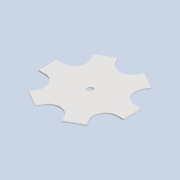
# Autodesk Inventor part: mid_7mm
Saved by Autodesk Inventor 2020 (Build 240168000, 168)
## iProperties
Created: 2021-10-03
Part Number: mid_7mm
Material: Generic
Document SubType Name: Modeling
Designer: Shuang Peng
Density: 1 g/cm^3
Appearance: Default
Author: Shuang Peng
Autodesk Inventor part; units mm, degrees
ref_plane "YZ Plane" through (0, 0, 0) normal (1, 0, 0) x (0, 1, 0)
ref_plane "XZ Plane" through (0, 0, 0) normal (0, 1, 0) x (-1, 0, 0)
ref_plane "XY Plane" through (0, 0, 0) normal (0, 0, 1) x (1, 0, 0)
sketch "Sketch1" plane through (0, 0, 0) normal (0, 1, 0) x (-1, 0, 0)
  circle A0 centre (0, 0) radius 1.5
  dimension "d0" = 3
  constraints: 1 centre point, 1 coincident
  measures "d0" diameter of A0
extrude "Extrusion1" add sketch "Sketch1" along normal blind 0.2
sketch "Sketch2" plane through (0, 0, 0) normal (0, 0, 1) x (1, 0, 0)
  line L0 (0, 0) -> (0, 0.1)
  line L1 (0, 0.1) -> (7, 0.1) construction
  line L2 (0, 0) -> (7, 0)
  line L3 (7, 0.2) -> (0, 0.2)
  arc A0 (0, 0.2) -> (0, 0) centre (0, 0.1) ccw
  arc A1 (7, 0) -> (7, 0.2) centre (7, 0.1) ccw
  line L4 (1.5, 0.2) -> (-1.5, 0.2) projected
  point P0 (3.5, 0.1)
  dimension "d3" = 0.1
  dimension "d4" = 7
  dimension "d5" = 0.2
  constraints: 10 end point, 4 point on circle, 4 tangent, 2 centre point, 1 collinear, 1 midpoint, 1 parallel, 1 vertical
  measures "d3" distance of L0.start L0.end
  measures "d4" distance of L0.end L1.end
  measures "d5" diameter of A1
extrude "Extrusion2" add sketch "Sketch2" along normal mid plane 3
pattern_circular "Circular Pattern1" count 6 over 360 about axis through (0, 0, 0) along (0, 1, 0) of "Extrusion2"
sketch "Sketch3" plane through (0, 0.2, 0) normal (0, 1, 0) x (1, 0, 0)
  circle A0 centre (0, 0) radius 0.5
  dimension "d11" = 1
  constraints: 1 centre point, 1 coincident
  measures "d11" diameter of A0
extrude "Extrusion3" cut sketch "Sketch3" against normal blind 1
fillet "Fillet1" radius 2 6 edges at (0, 0.1, -3) (-2.5981, 0.1, -1.5) (-2.5981, 0.1, 1.5) (0, 0.1, 3) (2.5981, 0.1, 1.5) (2.5981, 0.1, -1.5)
body "Solid1"
